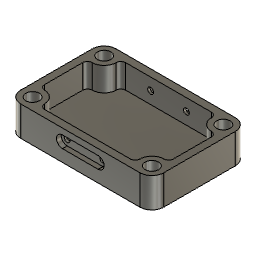
Engineering Drawings (Autodesk Fusion 360 design; units mm, degrees)
Autodesk Fusion 360 part; units mm, degrees
sketch "Sketch1" plane through (0, 0, 0) normal (0, 0, 1) x (1, 0, 0)
  line L0 (0, 0) -> (152.4, 0)
  line L1 (152.4, 0) -> (152.4, -101.6)
  line L2 (152.4, -101.6) -> (0, -101.6)
  line L3 (0, -101.6) -> (0, 0)
  dimension "d1" = 152.4
  dimension "d2" = 101.6
  constraint horizontal L0
  constraint vertical L1
  constraint horizontal L2
  constraint vertical L3
  constraint coincident L0.start L3.end
  measures "d1" distance of L0.start L0.end
  measures "d2" distance of L0.start L2.end
extrude "Extrude1" add sketch "Sketch1" along normal blind 31.75
fillet "Fillet1" radius 12.7 4 edges at (0, -101.6, 15.875) (152.4, -101.6, 15.875) (152.4, 0, 15.875) (0, 0, 15.875)
sketch "Sketch2" plane through (0, 0, 31.75) normal (0, 0, 1) x (-1, 0, 0)
  arc A0 (-12.7, 0) -> (0, 12.7) centre (-12.7, 12.7) ccw
  line L0 (0, 12.7) -> (0, 88.9)
  arc A1 (0, 88.9) -> (-12.7, 101.6) centre (-12.7, 88.9) ccw
  line L1 (-12.7, 101.6) -> (-139.7, 101.6)
  arc A2 (-139.7, 101.6) -> (-152.4, 88.9) centre (-139.7, 88.9) ccw
  line L2 (-152.4, 88.9) -> (-152.4, 12.7)
  arc A3 (-152.4, 12.7) -> (-139.7, 0) centre (-139.7, 12.7) ccw
  line L3 (-139.7, 0) -> (-12.7, 0)
  line L4 (-7.62, 12.7) -> (-7.62, 88.9)
  arc A4 (-7.62, 88.9) -> (-12.7, 93.98) centre (-12.7, 88.9) ccw
  line L5 (-12.7, 93.98) -> (-139.7, 93.98)
  arc A5 (-139.7, 93.98) -> (-144.78, 88.9) centre (-139.7, 88.9) ccw
  line L6 (-144.78, 88.9) -> (-144.78, 12.7)
  arc A6 (-144.78, 12.7) -> (-139.7, 7.62) centre (-139.7, 12.7) ccw
  line L7 (-139.7, 7.62) -> (-12.7, 7.62)
  arc A7 (-12.7, 7.62) -> (-7.62, 12.7) centre (-12.7, 12.7) ccw
  circle A8 centre (-12.7, 12.7) radius 12.7
  circle A9 centre (-139.7, 12.7) radius 12.7
  circle A10 centre (-139.7, 88.9) radius 12.7
  circle A11 centre (-12.7, 88.9) radius 12.7
  dimension "d7" = -7.62
  dimension "d8" = 25.4
  dimension "d9" = 25.4
  dimension "d10" = 25.4
  dimension "d11" = 25.4
  constraint concentric A0 A8
  constraint concentric A3 A9
  constraint concentric A2 A10
  constraint concentric A1 A11
  measures "d8" diameter of A8
  measures "d9" diameter of A9
  measures "d10" diameter of A10
  measures "d11" diameter of A11
extrude "Extrude2" cut sketch "Sketch2" against normal blind 25.4 contours L4 L5 L6 L7 A8 A9 A10 A11
fillet "Fillet2" radius 5.08 8 edges at (144.78, -24.3397, 19.05) (128.0603, -7.62, 19.05) (24.3397, -7.62, 19.05) (7.62, -24.3397, 19.05) (24.3397, -93.98, 19.05) (7.62, -77.2603, 19.05) (144.78, -77.2603, 19.05) (128.0603, -93.98, 19.05)
sketch "Sketch3" plane through (0, 0, 31.75) normal (0, 0, 1) x (-1, 0, 0)
  line L0 (-121.92, 93.98) -> (-30.48, 93.98)
  arc A0 (-25.4, 88.9) -> (-30.48, 93.98) centre (-30.48, 88.9) ccw
  arc A1 (-25.4, 88.9) -> (-12.7, 76.2) centre (-12.7, 88.9) ccw
  arc A2 (-7.62, 71.12) -> (-12.7, 76.2) centre (-12.7, 71.12) ccw
  line L1 (-7.62, 71.12) -> (-7.62, 30.48)
  arc A3 (-12.7, 25.4) -> (-7.62, 30.48) centre (-12.7, 30.48) ccw
  arc A4 (-12.7, 25.4) -> (-25.4, 12.7) centre (-12.7, 12.7) ccw
  arc A5 (-30.48, 7.62) -> (-25.4, 12.7) centre (-30.48, 12.7) ccw
  line L2 (-30.48, 7.62) -> (-121.92, 7.62)
  arc A6 (-127, 12.7) -> (-121.92, 7.62) centre (-121.92, 12.7) ccw
  arc A7 (-127, 12.7) -> (-139.7, 25.4) centre (-139.7, 12.7) ccw
  arc A8 (-144.78, 30.48) -> (-139.7, 25.4) centre (-139.7, 30.48) ccw
  line L3 (-144.78, 30.48) -> (-144.78, 71.12)
  arc A9 (-139.7, 76.2) -> (-144.78, 71.12) centre (-139.7, 71.12) ccw
  arc A10 (-139.7, 76.2) -> (-127, 88.9) centre (-139.7, 88.9) ccw
  arc A11 (-121.92, 93.98) -> (-127, 88.9) centre (-121.92, 88.9) ccw
  arc A12 (-12.7, 0) -> (0, 12.7) centre (-12.7, 12.7) ccw
  line L4 (0, 12.7) -> (0, 88.9)
  arc A13 (0, 88.9) -> (-12.7, 101.6) centre (-12.7, 88.9) ccw
  line L5 (-12.7, 101.6) -> (-139.7, 101.6)
  arc A14 (-139.7, 101.6) -> (-152.4, 88.9) centre (-139.7, 88.9) ccw
  line L6 (-152.4, 88.9) -> (-152.4, 12.7)
  arc A15 (-152.4, 12.7) -> (-139.7, 0) centre (-139.7, 12.7) ccw
  line L7 (-139.7, 0) -> (-12.7, 0)
  point P0 (-12.7, 88.9)
  point P1 (-12.7, 12.7)
  point P2 (-139.7, 12.7)
  point P3 (-139.7, 88.9)
  constraint coincident P0 A1.centre
  constraint coincident P1 A4.centre
  constraint coincident P2 A7.centre
  constraint coincident P3 A10.centre
hole "Hole1" at (12.7, -12.7, 31.75) at (139.7, -88.9, 31.75) at (139.7, -12.7, 31.75) at (12.7, -88.9, 31.75) direction (0, 0, -1) diameter 9.906 end through all counterbore diameter 14.224 counterbore depth 10.16
sketch "Sketch4" plane through (0, -101.6, 0) normal (0, -1, 0) x (1, 0, 0)
  line L0 (139.7, 0) -> (139.7, 31.75)
  line L1 (139.7, 31.75) -> (12.7, 31.75)
  line L2 (12.7, 31.75) -> (12.7, 0)
  line L3 (12.7, 0) -> (139.7, 0)
  line L4 (57.15, 12.7) -> (95.25, 12.7)
  arc A0 (95.25, 12.7) -> (95.25, 25.4) centre (95.25, 19.05) ccw
  line L5 (95.25, 25.4) -> (57.15, 25.4)
  arc A1 (57.15, 25.4) -> (57.15, 12.7) centre (57.15, 19.05) ccw
  line L6 (50.8, 19.05) -> (101.6, 19.05) construction
  line L7 (0, 31.75) -> (0, 0)
  circle A2 centre (57.15, 19.05) radius 3.175
  circle A3 centre (95.25, 19.05) radius 3.175
  point P0 (76.2, 19.05)
  dimension "d21" = 12.7
  dimension "d22" = 76.2
  dimension "d23" = 12.7
  dimension "d24" = 6.35
  dimension "d25" = 6.35
  constraint tangent L4 A0
  constraint tangent A0 L5
  constraint parallel L4 L5
  constraint tangent L5 A1
  constraint tangent L4 A1
  constraint midpoint A1 L6.start
  constraint midpoint A0 L6.end
  constraint parallel L3 L6
  constraint midpoint L6 P0
  constraint concentric A1 A2
  constraint concentric A0 A3
  measures "d21" diameter of A0
  measures "d22" distance of P0 L7
  measures "d23" distance of L1 P0
  measures "d24" diameter of A2
  measures "d25" diameter of A3
extrude "Extrude4" cut sketch "Sketch4" against normal blind 5.08 contours L4 A0 L5 A1
extrude "Extrude3" cut sketch "Sketch4" against normal through all contours A2 | A3
sketch "Sketch6" plane through (0, 0, 0) normal (0, 1, 0) x (-1, 0, 0)
  circle A0 centre (-57.15, 19.05) radius 3.175
  circle A1 centre (-95.25, 19.05) radius 3.175
  line L0 (-12.7, 0) -> (-12.7, 31.75)
  line L1 (-12.7, 31.75) -> (-139.7, 31.75)
  line L2 (-139.7, 31.75) -> (-139.7, 0)
  line L3 (-139.7, 0) -> (-12.7, 0)
  line L4 (-57.15, 25.4) -> (-95.25, 25.4)
  arc A2 (-95.25, 25.4) -> (-95.25, 12.7) centre (-95.25, 19.05) ccw
  line L5 (-95.25, 12.7) -> (-57.15, 12.7)
  arc A3 (-57.15, 12.7) -> (-57.15, 25.4) centre (-57.15, 19.05) ccw
  line L6 (-57.15, 19.05) -> (-95.25, 19.05) construction
  dimension "d29" = 12.7
  constraint tangent L4 A2
  constraint tangent A2 L5
  constraint parallel L4 L5
  constraint tangent L5 A3
  constraint tangent L4 A3
  constraint coincident A1.centre A2.centre
  constraint horizontal L6
  constraint coincident A0.centre A3.centre
  measures "d29" diameter of A2
extrude "Extrude5" cut sketch "Sketch6" against normal blind 5.08 contours L4 A2 L5 A3
equation "d25 = d24"
